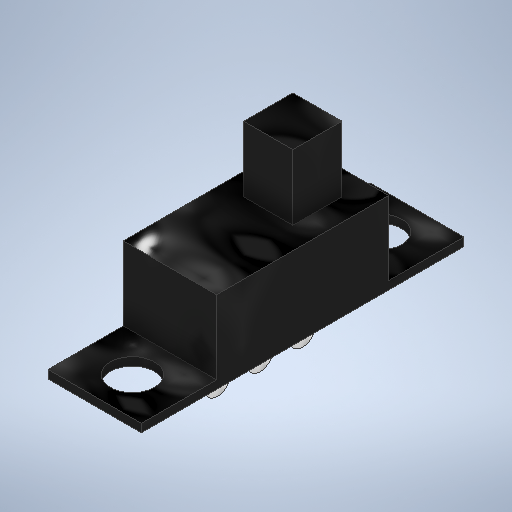
# Autodesk Inventor part: switch
Saved by Autodesk Inventor 2025.2 (Build 292293000, 293)
## iProperties
Created: 2025-06-11
Part Number: switch
Material: Generic
Document SubType Name: Modeling
Designer: cdavi
Density: 1 g/cm^3
Appearance: Default
Author: cdavi
Autodesk Inventor part; units mm, degrees
ref_plane "YZ Plane" through (0, 0, 0) normal (1, 0, 0) x (0, 1, 0)
ref_plane "XZ Plane" through (0, 0, 0) normal (0, 1, 0) x (-1, 0, 0)
ref_plane "XY Plane" through (0, 0, 0) normal (0, 0, 1) x (1, 0, 0)
sketch "Sketch1" plane through (0, 0, 0) normal (0, 1, 0) x (-1, 0, 0)
  line L0 (-2.85, 5.25) -> (2.85, 5.25)
  line L1 (2.85, 5.25) -> (2.85, -5.25)
  line L2 (2.85, -5.25) -> (-2.85, -5.25)
  line L3 (-2.85, -5.25) -> (-2.85, 5.25)
  line L4 (-2.85, 5.25) -> (2.85, -5.25) construction
  line L5 (2.85, 5.25) -> (-2.85, -5.25) construction
  line L6 (2.85, -5.25) -> (2.85, -9.85)
  line L7 (2.85, -9.85) -> (-2.85, -9.85)
  line L8 (-2.85, -9.85) -> (-2.85, -5.25)
  circle A0 centre (0, -7.55) radius 1.35
  line L9 (0, 0) -> (2.85, 0)
  line L10 (2.85, 5.25) -> (2.85, 9.85)
  line L11 (2.85, 9.85) -> (-2.85, 9.85)
  line L12 (-2.85, 9.85) -> (-2.85, 5.25)
  circle A1 centre (0, 7.55) radius 1.35
  point P0 (2.85, -7.55)
  point P1 (0, -9.85)
  point P2 (2.85, 7.55)
  point P3 (0, 9.85)
  dimension "d0" = 10.5
  dimension "d1" = 5.7
  dimension "d2" = 9.85
  dimension "d3" = 2.7
  constraints: 26 end point, 5 midpoint, 5 symmetric about line, 3 perpendicular, 2 centre point, 2 parallel, 1 horizontal, 1 horizontal alignment, 1 vertical, 1 vertical alignment, 1 other
  measures "d0" distance of L0.end L1.end
  measures "d1" distance of L1.end L2.end
  measures "d2" distance from line of L9.start L7
  measures "d3" diameter of A0
extrude "Extrusion1" add sketch "Sketch1" along normal blind 5 contours L0 L1 L2 L3
extrude "Extrusion2" add sketch "Sketch1" along normal blind 0.5 contours L12 L11 L10 L0 | L2 L6 L7 L8
sketch "Sketch2" plane through (0, 5, 0) normal (0, 1, 0) x (1, 0, 0)
  line L0 (1.5, 0.75) -> (-1.5, 0.75)
  line L1 (-1.5, 0.75) -> (-1.5, 3.75)
  line L2 (-1.5, 3.75) -> (1.5, 3.75)
  line L3 (1.5, 3.75) -> (1.5, 0.75)
  line L4 (1.5, 0.75) -> (-1.5, 3.75) construction
  line L5 (-1.5, 0.75) -> (1.5, 3.75) construction
  line L6 (2.85, 5.25) -> (-2.85, 5.25) projected
  point P0 (0, 0)
  point P1 (0, 2.25)
  dimension "d8" = 3
  dimension "d9" = 3
  dimension "d10" = 1.5
  constraints: 12 end point, 2 midpoint, 2 parallel, 1 horizontal, 1 perpendicular, 1 vertical alignment
  measures "d8" distance of L0.end L1.end
  measures "d9" distance of L0.start L0.end
  measures "d10" distance between parallel lines of L6 L2
extrude "Extrusion3" add sketch "Sketch2" along normal blind 4
sketch "Sketch3" plane through (0, 0, 0) normal (0, -1, 0) x (1, 0, 0)
  line L0 (0.25, 3.4) -> (-0.25, 3.4)
  line L1 (-0.25, 3.4) -> (-0.25, 1.8)
  line L2 (-0.25, 1.8) -> (0.25, 1.8)
  line L3 (0.25, 1.8) -> (0.25, 3.4)
  line L4 (0.25, 3.4) -> (-0.25, 1.8) construction
  line L5 (-0.25, 3.4) -> (0.25, 1.8) construction
  line L6 (-2.85, 5.25) -> (2.85, 5.25) projected
  line L7 (0.25, 0.8) -> (-0.25, 0.8)
  line L8 (-0.25, 0.8) -> (-0.25, -0.8)
  line L9 (-0.25, -0.8) -> (0.25, -0.8)
  line L10 (0.25, -0.8) -> (0.25, 0.8)
  line L11 (0.25, -1.8) -> (-0.25, -1.8)
  line L12 (-0.25, -1.8) -> (-0.25, -3.4)
  line L13 (-0.25, -3.4) -> (0.25, -3.4)
  line L14 (0.25, -3.4) -> (0.25, -1.8)
  line L15 (0.25, 0.8) -> (-0.25, -0.8)
  line L16 (-0.25, 0.8) -> (0.25, -0.8)
  point P0 (0, 0)
  point P1 (0, 2.6)
  point P2 (0, 0)
  dimension "d13" = 1.6
  dimension "d14" = 0.5
  dimension "d18" = 1.6
  dimension "d19" = 0.5
  dimension "d20" = 1.6
  dimension "d21" = 0.5
  dimension "d22" = 1
  dimension "d23" = 1
  constraints: 32 end point, 6 parallel, 3 horizontal, 3 midpoint, 3 perpendicular, 2 collinear, 1 coincident, 1 vertical alignment
  measures "d13" distance of L2.end L0.start
  measures "d14" distance of L1.end L2.end
  measures "d18" distance of L10.start L10.end
  measures "d19" distance of L9.start L10.start
  measures "d20" distance of L14.start L14.end
  measures "d21" distance of L13.start L14.start
  measures "d22" distance between parallel lines of L7 L2
  measures "d23" distance between parallel lines of L11 L9
extrude "Extrusion4" add sketch "Sketch3" along normal blind 3 separate body
full round fillet "Full Round Fillet1" bodies 2 first side at (0.0833, -1, 3.4) centre faces at (0.0833, -3, 2.3333) second side at (-0.0833, -1, 1.8)
full round fillet "Full Round Fillet2" bodies 2 first side at (0.0833, -1, 0.8) centre faces at (-0.0833, -3, 0.2667) second side at (-0.0833, -1, -0.8)
full round fillet "Full Round Fillet3" bodies 2 first side at (0.0833, -1, -1.8) centre faces at (0.0833, -3, -2.8667) second side at (-0.0833, -1, -3.4)
body "Solid1"
body "Solid2"
